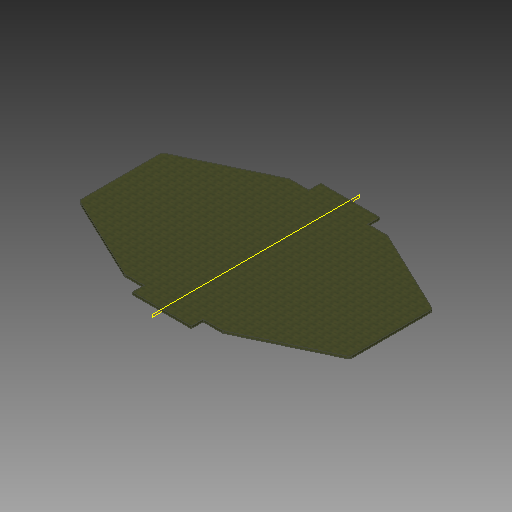
# Autodesk Inventor part: 1211_Racetrack Board_V1
Saved by Autodesk Inventor 2020 (Build 240168000, 168)
## iProperties
Created: 2017-06-05
Part Number: 1211_Racetrack Board_V1
Material: GFRP
Document SubType Name: Modeling
Designer: MPI
Density: 1.75 g/cm^3
Appearance: Smooth - Light Gray
Mass: 1509.01 g
Surface Area: 3702.26 cm^2
Volume: 862.293 cm^3
Author: MPI
Autodesk Inventor part; units mm, degrees
ref_plane "YZ Plane" through (0, 0, 0) normal (1, 0, 0) x (0, 1, 0)
ref_plane "XZ Plane" through (0, 0, 0) normal (0, 1, 0) x (-1, 0, 0)
sketch "Sketch1" plane through (0, 0, 0) normal (0, 0, 1) x (1, 0, 0)
  line L0 (42.4461, -373.0123) -> (525.0461, -373.0123)
  line L1 (575.8461, -322.2123) -> (575.8461, -68.2123) construction
  line L2 (525.0461, -17.4123) -> (42.4461, -17.4123)
  line L3 (-8.3539, -68.2123) -> (-8.3539, -322.2123) construction
  arc A0 (575.8461, -68.2123) -> (525.0461, -17.4123) centre (525.0461, -68.2123) ccw
  arc A1 (525.0461, -373.0123) -> (575.8461, -322.2123) centre (525.0461, -322.2123) ccw
  arc A2 (-8.3539, -322.2123) -> (42.4461, -373.0123) centre (42.4461, -322.2123) ccw
  arc A3 (42.4461, -17.4123) -> (-8.3539, -68.2123) centre (42.4461, -68.2123) ccw
  line L4 (-8.3539, -195.2123) -> (575.8461, -195.2123) construction
  line L5 (-8.3539, -106.3123) -> (177.9452, -17.4123)
  line L6 (-8.3539, -106.3123) -> (198.0693, -106.3123) construction
  line L7 (-8.3539, -284.1123) -> (177.9452, -373.0123)
  line L8 (283.7461, -17.4123) -> (283.7461, -373.0123) construction
  line L9 (575.8461, -106.3123) -> (389.5471, -17.4123)
  line L10 (575.8461, -284.1123) -> (389.5471, -373.0123)
  line L11 (575.8461, -106.3123) -> (575.8461, -284.1123)
  line L12 (-8.3539, -106.3123) -> (-8.3539, -284.1123)
  line L13 (177.9452, -17.4123) -> (389.5471, -17.4123)
  line L14 (389.5471, -373.0123) -> (177.9452, -373.0123)
  point P0 (0, 0)
  point P1 (-8.3539, -373.0123)
  point P2 (575.8461, -17.4123)
  point P3 (575.8461, -373.0123)
  point P4 (-8.3539, -17.4123)
  dimension "d0" = 355.6
  dimension "d1" = 584.2
  dimension "d4" = 50.8
  dimension "d25" = 25.51
  dimension "d26" = 254
  dimension "d27" = 88.9
  dimension "d28" = 575.8461
  dimension "d29" = 195.2123
  constraints: 30 end point, 12 point on line, 8 point on circle, 8 tangent, 6 symmetric about line, 4 centre point, 4 midpoint, 3 collinear, 3 equal radius, 3 horizontal, 2 parallel, 1 equal length, 1 perpendicular
  measures "d0" distance of point (-8.354, -17.412) point (-8.354, -373.012)
  measures "d1" distance of point (575.846, -17.412) point (-8.354, -17.412)
  measures "d4" radius of A0
  measures "d25" angle of L6 L5
  measures "d26" distance of L3.start L3.end
  measures "d27" distance between parallel lines of L2 L6
  measures "d28" distance from line of point (0, 0) L1
  measures "d29" distance from line of point (0, 0) L4
extrude "Extrusion1" add sketch "Sketch1" along normal blind 4.7625
sketch "Sketch2" plane through (0, 0, 0) normal (0, 0, 1) x (1, 0, 0)
  line L0 (283.7461, -373.0123) -> (347.2461, -373.0123)
  line L1 (347.2461, -373.0123) -> (347.2461, -398.4123)
  line L2 (347.2461, -398.4123) -> (283.7461, -398.4123)
  line L3 (220.2461, -373.0123) -> (347.2461, -373.0123)
  line L4 (347.2461, -373.0123) -> (347.2461, -398.4123)
  line L5 (347.2461, -398.4123) -> (220.2461, -398.4123)
  line L6 (220.2461, -398.4123) -> (220.2461, -373.0123)
  line L7 (220.2461, -373.0123) -> (347.2461, -398.4123) construction
  line L8 (347.2461, -373.0123) -> (220.2461, -398.4123) construction
  line L9 (283.7461, -17.4123) -> (347.2461, -17.4123)
  line L10 (347.2461, -17.4123) -> (347.2461, 7.9877)
  line L11 (347.2461, 7.9877) -> (283.7461, 7.9877)
  line L12 (220.2461, -17.4123) -> (347.2461, -17.4123)
  line L13 (347.2461, -17.4123) -> (347.2461, 7.9877)
  line L14 (347.2461, 7.9877) -> (220.2461, 7.9877)
  line L15 (220.2461, 7.9877) -> (220.2461, -17.4123)
  line L16 (220.2461, -17.4123) -> (347.2461, 7.9877) construction
  line L17 (347.2461, -17.4123) -> (220.2461, 7.9877) construction
  constraints: 36 end point, 2 parallel, 1 collinear, 1 perpendicular
extrude "Extrusion2" add sketch "Sketch2" along normal up to surface (4.7625 mm away)
fillet "Fillet1" radius 6 8 edges at (-8.3539, -106.3123, 2.3813) (-8.3539, -284.1123, 2.3813) (177.9452, -373.0123, 2.3813) (389.5471, -373.0123, 2.3813) (575.8461, -284.1123, 2.3813) (575.8461, -106.3123, 2.3813) (389.5471, -17.4123, 2.3813) (177.9452, -17.4123, 2.3813)
ref_plane "Work Plane1" through (220.2461, -195.2123, 0) normal (0, -1, 0) x (1, 0, 0)
ref_plane "Work Plane2" through (283.7461, -280.3273, 0) normal (1, 0, 0) x (0, 0, -1)
body "Solid1"
